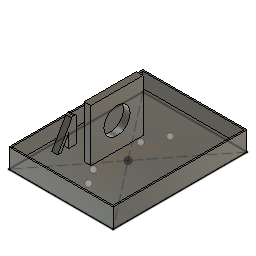
Single-throttle mount 1 (Autodesk Fusion 360 design; units mm, degrees)
Autodesk Fusion 360 part; units mm, degrees
sketch "Sketch1" plane through (0, 0, 0) normal (0, 0, 1) x (1, 0, 0)
  line L0 (35, 45) -> (-35, 45)
  line L1 (-35, 45) -> (-35, -45)
  line L2 (-35, -45) -> (35, -45)
  line L3 (35, -45) -> (35, 45)
  line L4 (35, 45) -> (-35, -45) construction
  line L5 (-35, 45) -> (35, -45) construction
  line L6 (0, 28.3109) -> (0, -26.5165) construction
  line L7 (-6.5, 15) -> (-6.5, -16.8183) construction
  dimension "d1" = 70
  dimension "d2" = 90
  dimension "d3" = 6.5
  constraint horizontal L0
  constraint perpendicular L0 L1
  constraint parallel L0 L2
  constraint parallel L1 L3
  constraint coincident L4 origin
  constraint coincident L5 origin
  constraint perpendicular L0 L6
  constraint perpendicular L0 L7
  measures "d1" distance of L1.end L2.end
  measures "d2" distance of L0.end L1.end
  measures "d3" distance of L6 L7
extrude "Extrude1" add sketch "Sketch1" along normal blind 3 makes body 1
sketch "Sketch2" plane through (0, 0, 3) normal (0, 0, 1) x (-1, 0, 0)
  line L0 (-35, 45) -> (-35, -45)
  line L1 (-35, -45) -> (35, -45)
  line L2 (35, -45) -> (35, 45)
  line L3 (35, 45) -> (-35, 45)
  line L4 (6.5, 18.4092) -> (11, 18.4092)
  line L5 (11, 18.4092) -> (11, -16.5908)
  line L6 (11, -16.5908) -> (6.5, -16.5908)
  line L7 (6.5, -16.5908) -> (6.5, 18.4092)
  line L8 (6.5, -15) -> (6.5, 16.8183)
  dimension "d6" = 4.5
  dimension "d7" = 35
  constraint horizontal L4
  constraint vertical L5
  constraint horizontal L6
  constraint vertical L7
  constraint midpoint L7 L8
  measures "d6" distance of L5 L7
  measures "d7" distance of L4 L6
extrude "Extrude2" add sketch "Sketch2" along normal blind 35 contours L4 L5 L6 L7 L8 bodies 1
sketch "Sketch3" plane through (0, 0, 3) normal (0, 0, 1) x (-1, 0, 0)
  line L0 (6.5, 18.4092) -> (11, 18.4092)
  line L1 (11, 18.4092) -> (11, -16.5908)
  line L2 (11, -16.5908) -> (6.5, -16.5908)
  line L3 (6.5, -16.5908) -> (6.5, 18.4092)
  line L4 (-35, 45) -> (-35, -45)
  line L5 (-35, -45) -> (35, -45)
  line L6 (35, -45) -> (35, 45)
  line L7 (35, 45) -> (-35, 45)
  line L8 (34, 44) -> (-34, 44)
  line L9 (-34, 44) -> (-34, -44)
  line L10 (-34, -44) -> (34, -44)
  line L11 (34, -44) -> (34, 44)
  line L12 (34, 44) -> (-34, -44) construction
  line L13 (-34, 44) -> (34, -44) construction
  dimension "d10" = 68
  dimension "d11" = 88
  constraint horizontal L8
  constraint perpendicular L8 L9
  constraint parallel L8 L10
  constraint parallel L9 L11
  constraint coincident L12 origin
  constraint coincident L13 origin
  measures "d10" distance of L9.end L10.end
  measures "d11" distance of L8.end L9.end
extrude "Extrude3" add sketch "Sketch3" along normal blind 10 contours L4 L5 L6 L7 bodies 1
sketch "Sketch4" plane through (-11, 0, 0) normal (-1, 0, 0) x (0, -1, 0)
  line L0 (-16.5908, 3) -> (18.4092, 3)
  line L1 (18.4092, 3) -> (18.4092, 38)
  line L2 (18.4092, 38) -> (-16.5908, 38)
  line L3 (-16.5908, 38) -> (-16.5908, 3)
  circle A0 centre (0.9092, 20.5) radius 8.8
  line L4 (-16.5908, 3) -> (-16.5908, 38)
  line L5 (-16.5908, 38) -> (18.4092, 38)
  line L6 (18.4092, 3) -> (18.4092, 38)
  line L7 (18.4092, 3) -> (-16.5908, 3)
  line L8 (-16.5908, 38) -> (18.4092, 3) construction
  line L9 (10.9092, 3) -> (13.7611, 3)
  line L10 (13.7611, 3) -> (13.7611, 19.5)
  line L11 (12.7611, 20.5) -> (11.9092, 20.5)
  line L12 (10.9092, 19.5) -> (10.9092, 3)
  line L13 (-5.4652, 20.5) -> (30.4752, 20.5) construction
  arc A1 (11.9092, 20.5) -> (10.9092, 19.5) centre (11.9092, 19.5) ccw
  arc A2 (13.7611, 19.5) -> (12.7611, 20.5) centre (12.7611, 19.5) ccw
  dimension "d14" = 17.6
  dimension "d15" = 10
  dimension "d16" = 1
  constraint coincident L2.end L3.start
  constraint coincident L0.end L1.start
  constraint midpoint A0.centre L8
  constraint horizontal L9
  constraint vertical L10
  constraint horizontal L11
  constraint vertical L12
  constraint collinear L0 L9
  constraint perpendicular L6 L13
  constraint collinear L11 L13
  constraint coincident A0.centre L13
  constraint tangent L11 A1
  constraint tangent L12 A1
  constraint tangent L10 A2
  constraint tangent L11 A2
  constraint equal A1 A2
  measures "d14" diameter of A0
  measures "d15" distance of A0.centre L12
  measures "d16" radius of A1
extrude "Extrude4" add sketch "Sketch4" along normal blind 4 separate body contours L0 L7 L9 L10 L11 L12 A1 A2 makes body 2
move_body "Move1" bodies 2 to x (1, 0, 0) y (0, 1, 0) z (0, 0, 1) at (-13, 0, 0)
sketch "Sketch5" plane through (-28, 0, 0) normal (-1, 0, 0) x (0, -1, 0)
  arc A0 (13.7611, 19.5) -> (12.7611, 20.5) centre (12.7611, 19.5) ccw
  line L0 (12.7611, 20.5) -> (11.9092, 20.5)
  arc A1 (11.9092, 20.5) -> (10.9092, 19.5) centre (11.9092, 19.5) ccw
  line L1 (10.9092, 19.5) -> (10.9092, 3)
  line L2 (10.9092, 3) -> (13.7611, 3)
  line L3 (13.7611, 3) -> (13.7611, 19.5)
  line L4 (13.7611, 19.5) -> (23.2874, 3)
  line L5 (13.7611, 19.5) -> (32.9491, 19.5) construction
  line L6 (23.2874, 3) -> (10.9092, 3)
  line L7 (13.7611, 19.5) -> (13.7611, 3)
  line L8 (15.7611, 12.0359) -> (21.5554, 2)
  line L9 (15.7611, 12.0359) -> (15.7611, 3)
  dimension "d19" = 60
  dimension "d20" = -2
  constraint horizontal L5
  constraint coincident A0.start L3.end
  constraint coincident L1.end L2.start
  constraint horizontal L6
  constraint coincident L2.end L3.start
  measures "d19" angle of L4 L5
extrude "Extrude5" add sketch "Sketch5" against normal blind 4 contours L3 L4 L6 L7 L8 L9 bodies 1 2
extrude "Extrude6" cut sketch "Sketch4" against normal blind 6 contours A0 bodies 1
